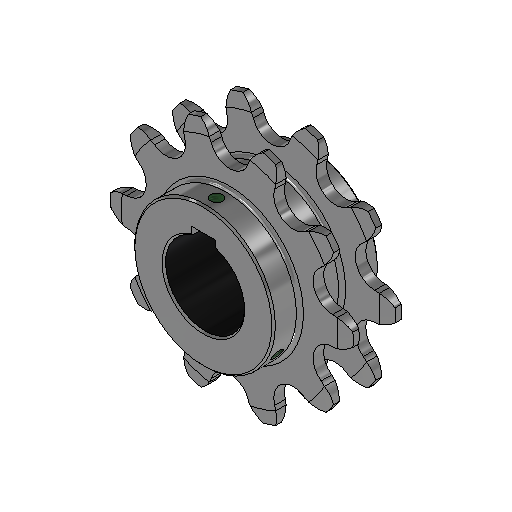
# Autodesk Inventor part: TL20240701-10110CV-016
Saved by Autodesk Inventor 2022.5 (Build 265521000, 521)
## iProperties
Category: DRIVE UNIT ASSY
Manager: 호상태
Company: 현대 트랜시스(대유)
Created: 2023-01-19
Part Number: TL20240701-10110CV-016
Project: SW PJT
Checked By: 김형민
Engr Approved By: 김시현
User Status: 2 x18
Material: S45C
Description: 0
Document SubType Name: Modeling
Mfg Approved By: 호상태
Designer: 박성규
Stock Number: 016
Density: 7.87 g/cm^3
Appearance: Plating Chrome
DETAIL: Coveryor Assembly
M/C TITLE: MEa/NEa차종 시트조립라인
SPECIFICATION: TL20221201-000000CV-006
DocNumber: 221118_Standard_v1
Folder: .\
VDS_Category: 엔지니어링
Detail Description: Processed products
Title: SPROCKET
Subject: SW차종 시트조립라인
Author: 박성규
Comments: RF2060 10NT
Revision Number: A
Autodesk Inventor part; units mm, degrees
ref_plane "YZ Plane" through (0, 0, 0) normal (1, 0, 0) x (0, 1, 0)
ref_plane "XZ Plane" through (0, 0, 0) normal (0, 1, 0) x (-1, 0, 0)
ref_plane "XY Plane" through (0, 0, 0) normal (0, 0, 1) x (1, 0, 0)
sketch "스케치8" plane through (0, 0, 0) normal (0, 0, 1) x (1, 0, 0)
  spline S0 degree 3 poles (-26.1552, 55.8268) (-26.2325, 56.5011) (-26.2682, 57.1822) (-26.249, 59.154) (-26.0828, 60.4461) (-25.5414, 62.6157) (-25.2309, 63.515) (-24.853, 64.3687) knots 0.551203 0.551203 0.551203 0.551203 0.748529 0.748529 1.122794 1.122794 1.401532 1.401532 1.401532 1.401532
  line L0 (-26.1552, 55.8268) -> (-26.2325, 56.5011) construction
  line L1 (-26.2325, 56.5011) -> (-26.2682, 57.1822) construction
  line L2 (-26.2682, 57.1822) -> (-26.249, 59.154) construction
  line L3 (-26.249, 59.154) -> (-26.0828, 60.4461) construction
  line L4 (-26.0828, 60.4461) -> (-25.5414, 62.6157) construction
  line L5 (-25.5414, 62.6157) -> (-25.2309, 63.515) construction
  line L6 (-25.2309, 63.515) -> (-24.853, 64.3687) construction
  arc A0 (-17.7285, 66.6836) -> (-24.853, 64.3687) centre (0, 0) ccw
  spline S1 degree 3 poles (-17.7285, 66.6836) (-16.921, 66.215) (-16.1411, 65.67) (-14.4279, 64.233) (-13.5339, 63.2854) (-12.3594, 61.7015) (-11.9879, 61.1294) (-11.6541, 60.5384) knots 4.560607 4.560607 4.560607 4.560607 4.839345 4.839345 5.213609 5.213609 5.410936 5.410936 5.410936 5.410936
  line L7 (-17.7285, 66.6836) -> (-16.921, 66.215) construction
  line L8 (-16.921, 66.215) -> (-16.1411, 65.67) construction
  line L9 (-16.1411, 65.67) -> (-14.4279, 64.233) construction
  line L10 (-14.4279, 64.233) -> (-13.5339, 63.2854) construction
  line L11 (-13.5339, 63.2854) -> (-12.3594, 61.7015) construction
  line L12 (-12.3594, 61.7015) -> (-11.9879, 61.1294) construction
  line L13 (-11.9879, 61.1294) -> (-11.6541, 60.5384) construction
  spline S2 degree 3 poles (11.6541, 60.5384) (11.9879, 61.1294) (12.3594, 61.7015) (13.5339, 63.2854) (14.4279, 64.233) (16.1411, 65.67) (16.921, 66.215) (17.7285, 66.6836) knots 0.551203 0.551203 0.551203 0.551203 0.748529 0.748529 1.122794 1.122794 1.401532 1.401532 1.401532 1.401532
  line L14 (11.6541, 60.5384) -> (11.9879, 61.1294) construction
  line L15 (11.9879, 61.1294) -> (12.3594, 61.7015) construction
  line L16 (12.3594, 61.7015) -> (13.5339, 63.2854) construction
  line L17 (13.5339, 63.2854) -> (14.4279, 64.233) construction
  line L18 (14.4279, 64.233) -> (16.1411, 65.67) construction
  line L19 (16.1411, 65.67) -> (16.921, 66.215) construction
  line L20 (16.921, 66.215) -> (17.7285, 66.6836) construction
  arc A1 (24.853, 64.3687) -> (17.7285, 66.6836) centre (0, 0) ccw
  spline S3 degree 3 poles (24.853, 64.3687) (25.2309, 63.515) (25.5414, 62.6157) (26.0828, 60.4461) (26.249, 59.154) (26.2682, 57.1822) (26.2325, 56.5011) (26.1552, 55.8268) knots 4.560607 4.560607 4.560607 4.560607 4.839345 4.839345 5.213609 5.213609 5.410936 5.410936 5.410936 5.410936
  line L21 (24.853, 64.3687) -> (25.2309, 63.515) construction
  line L22 (25.2309, 63.515) -> (25.5414, 62.6157) construction
  line L23 (25.5414, 62.6157) -> (26.0828, 60.4461) construction
  line L24 (26.0828, 60.4461) -> (26.249, 59.154) construction
  line L25 (26.249, 59.154) -> (26.2682, 57.1822) construction
  line L26 (26.2682, 57.1822) -> (26.2325, 56.5011) construction
  line L27 (26.2325, 56.5011) -> (26.1552, 55.8268) construction
  spline S4 degree 3 poles (45.012, 42.1265) (45.6294, 42.4084) (46.2662, 42.6528) (48.1474, 43.2439) (49.4276, 43.485) (51.6583, 43.6406) (52.6096, 43.6232) (53.5383, 43.5276) knots 0.551203 0.551203 0.551203 0.551203 0.748529 0.748529 1.122794 1.122794 1.401532 1.401532 1.401532 1.401532
  line L28 (45.012, 42.1265) -> (45.6294, 42.4084) construction
  line L29 (45.6294, 42.4084) -> (46.2662, 42.6528) construction
  line L30 (46.2662, 42.6528) -> (48.1474, 43.2439) construction
  line L31 (48.1474, 43.2439) -> (49.4276, 43.485) construction
  line L32 (49.4276, 43.485) -> (51.6583, 43.6406) construction
  line L33 (51.6583, 43.6406) -> (52.6096, 43.6232) construction
  line L34 (52.6096, 43.6232) -> (53.5383, 43.5276) construction
  arc A2 (57.9415, 37.4671) -> (53.5383, 43.5276) centre (0, 0) ccw
  spline S5 degree 3 poles (57.9415, 37.4671) (57.7454, 36.5544) (57.468, 35.6443) (56.6307, 33.5708) (56.0057, 32.4278) (54.8623, 30.8213) (54.433, 30.2912) (53.9742, 29.7912) knots 4.560607 4.560607 4.560607 4.560607 4.839345 4.839345 5.213609 5.213609 5.410936 5.410936 5.410936 5.410936
  line L35 (57.9415, 37.4671) -> (57.7454, 36.5544) construction
  line L36 (57.7454, 36.5544) -> (57.468, 35.6443) construction
  line L37 (57.468, 35.6443) -> (56.6307, 33.5708) construction
  line L38 (56.6307, 33.5708) -> (56.0057, 32.4278) construction
  line L39 (56.0057, 32.4278) -> (54.8623, 30.8213) construction
  line L40 (54.8623, 30.8213) -> (54.433, 30.2912) construction
  line L41 (54.433, 30.2912) -> (53.9742, 29.7912) construction
  spline S6 degree 3 poles (61.1768, 7.6237) (61.842, 7.4888) (62.5009, 7.3123) (64.3702, 6.6847) (65.5477, 6.1273) (67.4438, 4.942) (68.2031, 4.3688) (68.8983, 3.7456) knots 0.551203 0.551203 0.551203 0.551203 0.748529 0.748529 1.122794 1.122794 1.401532 1.401532 1.401532 1.401532
  line L42 (61.1768, 7.6237) -> (61.842, 7.4888) construction
  line L43 (61.842, 7.4888) -> (62.5009, 7.3123) construction
  line L44 (62.5009, 7.3123) -> (64.3702, 6.6847) construction
  line L45 (64.3702, 6.6847) -> (65.5477, 6.1273) construction
  line L46 (65.5477, 6.1273) -> (67.4438, 4.942) construction
  line L47 (67.4438, 4.942) -> (68.2031, 4.3688) construction
  line L48 (68.2031, 4.3688) -> (68.8983, 3.7456) construction
  arc A3 (68.8983, -3.7456) -> (68.8983, 3.7456) centre (0, 0) ccw
  spline S7 degree 3 poles (68.8983, -3.7456) (68.2031, -4.3688) (67.4438, -4.942) (65.5477, -6.1273) (64.3702, -6.6847) (62.5009, -7.3123) (61.842, -7.4888) (61.1768, -7.6237) knots 4.560607 4.560607 4.560607 4.560607 4.839345 4.839345 5.213609 5.213609 5.410936 5.410936 5.410936 5.410936
  line L49 (68.8983, -3.7456) -> (68.2031, -4.3688) construction
  line L50 (68.2031, -4.3688) -> (67.4438, -4.942) construction
  line L51 (67.4438, -4.942) -> (65.5477, -6.1273) construction
  line L52 (65.5477, -6.1273) -> (64.3702, -6.6847) construction
  line L53 (64.3702, -6.6847) -> (62.5009, -7.3123) construction
  line L54 (62.5009, -7.3123) -> (61.842, -7.4888) construction
  line L55 (61.842, -7.4888) -> (61.1768, -7.6237) construction
  spline S8 degree 3 poles (53.9742, -29.7912) (54.433, -30.2912) (54.8623, -30.8213) (56.0057, -32.4278) (56.6307, -33.5708) (57.468, -35.6443) (57.7454, -36.5544) (57.9415, -37.4671) knots 0.551203 0.551203 0.551203 0.551203 0.748529 0.748529 1.122794 1.122794 1.401532 1.401532 1.401532 1.401532
  line L56 (53.9742, -29.7912) -> (54.433, -30.2912) construction
  line L57 (54.433, -30.2912) -> (54.8623, -30.8213) construction
  line L58 (54.8623, -30.8213) -> (56.0057, -32.4278) construction
  line L59 (56.0057, -32.4278) -> (56.6307, -33.5708) construction
  line L60 (56.6307, -33.5708) -> (57.468, -35.6443) construction
  line L61 (57.468, -35.6443) -> (57.7454, -36.5544) construction
  line L62 (57.7454, -36.5544) -> (57.9415, -37.4671) construction
  arc A4 (53.5383, -43.5276) -> (57.9415, -37.4671) centre (0, 0) ccw
  spline S9 degree 3 poles (53.5383, -43.5276) (52.6096, -43.6232) (51.6583, -43.6406) (49.4276, -43.485) (48.1474, -43.2439) (46.2662, -42.6528) (45.6294, -42.4084) (45.012, -42.1265) knots 4.560607 4.560607 4.560607 4.560607 4.839345 4.839345 5.213609 5.213609 5.410936 5.410936 5.410936 5.410936
  line L63 (53.5383, -43.5276) -> (52.6096, -43.6232) construction
  line L64 (52.6096, -43.6232) -> (51.6583, -43.6406) construction
  line L65 (51.6583, -43.6406) -> (49.4276, -43.485) construction
  line L66 (49.4276, -43.485) -> (48.1474, -43.2439) construction
  line L67 (48.1474, -43.2439) -> (46.2662, -42.6528) construction
  line L68 (46.2662, -42.6528) -> (45.6294, -42.4084) construction
  line L69 (45.6294, -42.4084) -> (45.012, -42.1265) construction
  spline S10 degree 3 poles (26.1552, -55.8268) (26.2325, -56.5011) (26.2682, -57.1822) (26.249, -59.154) (26.0828, -60.4461) (25.5414, -62.6157) (25.2309, -63.515) (24.853, -64.3687) knots 0.551203 0.551203 0.551203 0.551203 0.748529 0.748529 1.122794 1.122794 1.401532 1.401532 1.401532 1.401532
  line L70 (26.1552, -55.8268) -> (26.2325, -56.5011) construction
  line L71 (26.2325, -56.5011) -> (26.2682, -57.1822) construction
  line L72 (26.2682, -57.1822) -> (26.249, -59.154) construction
  line L73 (26.249, -59.154) -> (26.0828, -60.4461) construction
  line L74 (26.0828, -60.4461) -> (25.5414, -62.6157) construction
  line L75 (25.5414, -62.6157) -> (25.2309, -63.515) construction
  line L76 (25.2309, -63.515) -> (24.853, -64.3687) construction
  arc A5 (17.7285, -66.6836) -> (24.853, -64.3687) centre (0, 0) ccw
  spline S11 degree 3 poles (17.7285, -66.6836) (16.921, -66.215) (16.1411, -65.67) (14.4279, -64.233) (13.5339, -63.2854) (12.3594, -61.7015) (11.9879, -61.1294) (11.6541, -60.5384) knots 4.560607 4.560607 4.560607 4.560607 4.839345 4.839345 5.213609 5.213609 5.410936 5.410936 5.410936 5.410936
  line L77 (17.7285, -66.6836) -> (16.921, -66.215) construction
  line L78 (16.921, -66.215) -> (16.1411, -65.67) construction
  line L79 (16.1411, -65.67) -> (14.4279, -64.233) construction
  line L80 (14.4279, -64.233) -> (13.5339, -63.2854) construction
  line L81 (13.5339, -63.2854) -> (12.3594, -61.7015) construction
  line L82 (12.3594, -61.7015) -> (11.9879, -61.1294) construction
  line L83 (11.9879, -61.1294) -> (11.6541, -60.5384) construction
  spline S12 degree 3 poles (-11.6541, -60.5384) (-11.9879, -61.1294) (-12.3594, -61.7015) (-13.5339, -63.2854) (-14.4279, -64.233) (-16.1411, -65.67) (-16.921, -66.215) (-17.7285, -66.6836) knots 0.551203 0.551203 0.551203 0.551203 0.748529 0.748529 1.122794 1.122794 1.401532 1.401532 1.401532 1.401532
  line L84 (-11.6541, -60.5384) -> (-11.9879, -61.1294) construction
  line L85 (-11.9879, -61.1294) -> (-12.3594, -61.7015) construction
  line L86 (-12.3594, -61.7015) -> (-13.5339, -63.2854) construction
  line L87 (-13.5339, -63.2854) -> (-14.4279, -64.233) construction
  line L88 (-14.4279, -64.233) -> (-16.1411, -65.67) construction
  line L89 (-16.1411, -65.67) -> (-16.921, -66.215) construction
  line L90 (-16.921, -66.215) -> (-17.7285, -66.6836) construction
  arc A6 (-24.853, -64.3687) -> (-17.7285, -66.6836) centre (0, 0) ccw
  spline S13 degree 3 poles (-24.853, -64.3687) (-25.2309, -63.515) (-25.5414, -62.6157) (-26.0828, -60.4461) (-26.249, -59.154) (-26.2682, -57.1822) (-26.2325, -56.5011) (-26.1552, -55.8268) knots 4.560607 4.560607 4.560607 4.560607 4.839345 4.839345 5.213609 5.213609 5.410936 5.410936 5.410936 5.410936
  line L91 (-24.853, -64.3687) -> (-25.2309, -63.515) construction
  line L92 (-25.2309, -63.515) -> (-25.5414, -62.6157) construction
  line L93 (-25.5414, -62.6157) -> (-26.0828, -60.4461) construction
  line L94 (-26.0828, -60.4461) -> (-26.249, -59.154) construction
  line L95 (-26.249, -59.154) -> (-26.2682, -57.1822) construction
  line L96 (-26.2682, -57.1822) -> (-26.2325, -56.5011) construction
  line L97 (-26.2325, -56.5011) -> (-26.1552, -55.8268) construction
  spline S14 degree 3 poles (-45.012, -42.1265) (-45.6294, -42.4084) (-46.2662, -42.6528) (-48.1474, -43.2439) (-49.4276, -43.485) (-51.6583, -43.6406) (-52.6096, -43.6232) (-53.5383, -43.5276) knots 0.551203 0.551203 0.551203 0.551203 0.748529 0.748529 1.122794 1.122794 1.401532 1.401532 1.401532 1.401532
  line L98 (-45.012, -42.1265) -> (-45.6294, -42.4084) construction
  line L99 (-45.6294, -42.4084) -> (-46.2662, -42.6528) construction
  line L100 (-46.2662, -42.6528) -> (-48.1474, -43.2439) construction
  line L101 (-48.1474, -43.2439) -> (-49.4276, -43.485) construction
  line L102 (-49.4276, -43.485) -> (-51.6583, -43.6406) construction
  line L103 (-51.6583, -43.6406) -> (-52.6096, -43.6232) construction
  line L104 (-52.6096, -43.6232) -> (-53.5383, -43.5276) construction
  arc A7 (-57.9415, -37.4671) -> (-53.5383, -43.5276) centre (0, 0) ccw
  spline S15 degree 3 poles (-57.9415, -37.4671) (-57.7454, -36.5544) (-57.468, -35.6443) (-56.6307, -33.5708) (-56.0057, -32.4278) (-54.8623, -30.8213) (-54.433, -30.2912) (-53.9742, -29.7912) knots 4.560607 4.560607 4.560607 4.560607 4.839345 4.839345 5.213609 5.213609 5.410936 5.410936 5.410936 5.410936
  line L105 (-57.9415, -37.4671) -> (-57.7454, -36.5544) construction
  line L106 (-57.7454, -36.5544) -> (-57.468, -35.6443) construction
  line L107 (-57.468, -35.6443) -> (-56.6307, -33.5708) construction
  line L108 (-56.6307, -33.5708) -> (-56.0057, -32.4278) construction
  line L109 (-56.0057, -32.4278) -> (-54.8623, -30.8213) construction
  line L110 (-54.8623, -30.8213) -> (-54.433, -30.2912) construction
  line L111 (-54.433, -30.2912) -> (-53.9742, -29.7912) construction
  spline S16 degree 3 poles (-53.9742, 29.7912) (-54.433, 30.2912) (-54.8623, 30.8213) (-56.0057, 32.4278) (-56.6307, 33.5708) (-57.468, 35.6443) (-57.7454, 36.5544) (-57.9415, 37.4671) knots 0.551203 0.551203 0.551203 0.551203 0.748529 0.748529 1.122794 1.122794 1.401532 1.401532 1.401532 1.401532
  line L112 (-53.9742, 29.7912) -> (-54.433, 30.2912) construction
  line L113 (-54.433, 30.2912) -> (-54.8623, 30.8213) construction
  line L114 (-54.8623, 30.8213) -> (-56.0057, 32.4278) construction
  line L115 (-56.0057, 32.4278) -> (-56.6307, 33.5708) construction
  line L116 (-56.6307, 33.5708) -> (-57.468, 35.6443) construction
  line L117 (-57.468, 35.6443) -> (-57.7454, 36.5544) construction
  line L118 (-57.7454, 36.5544) -> (-57.9415, 37.4671) construction
  arc A8 (-53.5383, 43.5276) -> (-57.9415, 37.4671) centre (0, 0) ccw
  spline S17 degree 3 poles (-53.5383, 43.5276) (-52.6096, 43.6232) (-51.6583, 43.6406) (-49.4276, 43.485) (-48.1474, 43.2439) (-46.2662, 42.6528) (-45.6294, 42.4084) (-45.012, 42.1265) knots 4.560607 4.560607 4.560607 4.560607 4.839345 4.839345 5.213609 5.213609 5.410936 5.410936 5.410936 5.410936
  line L119 (-53.5383, 43.5276) -> (-52.6096, 43.6232) construction
  line L120 (-52.6096, 43.6232) -> (-51.6583, 43.6406) construction
  line L121 (-51.6583, 43.6406) -> (-49.4276, 43.485) construction
  line L122 (-49.4276, 43.485) -> (-48.1474, 43.2439) construction
  line L123 (-48.1474, 43.2439) -> (-46.2662, 42.6528) construction
  line L124 (-46.2662, 42.6528) -> (-45.6294, 42.4084) construction
  line L125 (-45.6294, 42.4084) -> (-45.012, 42.1265) construction
  spline S18 degree 3 poles (-68.8983, 3.7456) (-68.2031, 4.3688) (-67.4438, 4.942) (-65.5477, 6.1273) (-64.3702, 6.6847) (-62.5009, 7.3123) (-61.842, 7.4888) (-61.1768, 7.6237) knots 4.560607 4.560607 4.560607 4.560607 4.839345 4.839345 5.213609 5.213609 5.410936 5.410936 5.410936 5.410936
  line L126 (-68.8983, 3.7456) -> (-68.2031, 4.3688) construction
  line L127 (-68.2031, 4.3688) -> (-67.4438, 4.942) construction
  line L128 (-67.4438, 4.942) -> (-65.5477, 6.1273) construction
  line L129 (-65.5477, 6.1273) -> (-64.3702, 6.6847) construction
  line L130 (-64.3702, 6.6847) -> (-62.5009, 7.3123) construction
  line L131 (-62.5009, 7.3123) -> (-61.842, 7.4888) construction
  line L132 (-61.842, 7.4888) -> (-61.1768, 7.6237) construction
  spline S19 degree 3 poles (-61.1768, -7.6237) (-61.842, -7.4888) (-62.5009, -7.3123) (-64.3702, -6.6847) (-65.5477, -6.1273) (-67.4438, -4.942) (-68.2031, -4.3688) (-68.8983, -3.7456) knots 0.551203 0.551203 0.551203 0.551203 0.748529 0.748529 1.122794 1.122794 1.401532 1.401532 1.401532 1.401532
  line L133 (-61.1768, -7.6237) -> (-61.842, -7.4888) construction
  line L134 (-61.842, -7.4888) -> (-62.5009, -7.3123) construction
  line L135 (-62.5009, -7.3123) -> (-64.3702, -6.6847) construction
  line L136 (-64.3702, -6.6847) -> (-65.5477, -6.1273) construction
  line L137 (-65.5477, -6.1273) -> (-67.4438, -4.942) construction
  line L138 (-67.4438, -4.942) -> (-68.2031, -4.3688) construction
  line L139 (-68.2031, -4.3688) -> (-68.8983, -3.7456) construction
  arc A9 (-68.8983, 3.7456) -> (-68.8983, -3.7456) centre (0, 0) ccw
  arc A10 (45.012, 42.1265) -> (42.7702, 40.8837) centre (51.8522, 27.1447) ccw
  arc A11 (11.6541, 60.5384) -> (10.571, 58.2153) centre (25.9941, 52.4385) ccw
  arc A12 (-26.1552, 55.8268) -> (-25.666, 53.3106) centre (-9.7929, 57.7026) ccw
  arc A13 (-53.9742, 29.7912) -> (-52.0994, 28.0431) centre (-41.8394, 40.9262) ccw
  arc A14 (-45.012, -42.1265) -> (-42.7702, -40.8837) centre (-51.8522, -27.1447) ccw
  arc A15 (-11.6541, -60.5384) -> (-10.571, -58.2153) centre (-25.9941, -52.4385) ccw
  arc A16 (26.1552, -55.8268) -> (25.666, -53.3106) centre (9.7929, -57.7026) ccw
  arc A17 (53.9742, -29.7912) -> (52.0994, -28.0431) centre (41.8394, -40.9262) ccw
  arc A18 (61.1768, 7.6237) -> (58.6326, 7.9359) centre (57.9046, -8.5175) ccw
  arc A19 (-58.6326, 7.9359) -> (-61.1768, 7.6237) centre (-57.9046, -8.5175) ccw
  arc A20 (-58.6326, 7.9359) -> (-52.0994, 28.0431) centre (-58.6326, 19.0509) ccw
  arc A21 (-42.7702, 40.8837) -> (-45.012, 42.1265) centre (-51.8522, 27.1447) ccw
  arc A22 (-42.7702, 40.8837) -> (-25.666, 53.3106) centre (-36.237, 49.8759) ccw
  arc A23 (-10.571, 58.2153) -> (-11.6541, 60.5384) centre (-25.9941, 52.4385) ccw
  arc A24 (-10.571, 58.2153) -> (10.571, 58.2153) centre (0, 61.65) ccw
  arc A25 (25.666, 53.3106) -> (26.1552, 55.8268) centre (9.7929, 57.7026) ccw
  arc A26 (25.666, 53.3106) -> (42.7702, 40.8837) centre (36.237, 49.8759) ccw
  arc A27 (52.0994, 28.0431) -> (53.9742, 29.7912) centre (41.8394, 40.9262) ccw
  arc A28 (52.0994, 28.0431) -> (58.6326, 7.9359) centre (58.6326, 19.0509) ccw
  arc A29 (58.6326, -7.9359) -> (61.1768, -7.6237) centre (57.9046, 8.5175) ccw
  arc A30 (58.6326, -7.9359) -> (52.0994, -28.0431) centre (58.6326, -19.0509) ccw
  arc A31 (42.7702, -40.8837) -> (45.012, -42.1265) centre (51.8522, -27.1447) ccw
  arc A32 (42.7702, -40.8837) -> (25.666, -53.3106) centre (36.237, -49.8759) ccw
  arc A33 (10.571, -58.2153) -> (11.6541, -60.5384) centre (25.9941, -52.4385) ccw
  arc A34 (10.571, -58.2153) -> (-10.571, -58.2153) centre (0, -61.65) ccw
  arc A35 (-25.666, -53.3106) -> (-26.1552, -55.8268) centre (-9.7929, -57.7026) ccw
  arc A36 (-25.666, -53.3106) -> (-42.7702, -40.8837) centre (-36.237, -49.8759) ccw
  arc A37 (-52.0994, -28.0431) -> (-53.9742, -29.7912) centre (-41.8394, -40.9262) ccw
  arc A38 (-52.0994, -28.0431) -> (-58.6326, -7.9359) centre (-58.6326, -19.0509) ccw
  arc A39 (-61.1768, -7.6237) -> (-58.6326, -7.9359) centre (-57.9046, 8.5175) ccw
  point P0 (0, 0)
  constraints: 80 point on circle, 40 centre point, 1 coincident, 60 other
extrude "돌출3" add sketch "스케치8" along normal blind 6
sketch "스케치9" plane through (0, 0, 6) normal (0, 0, 1) x (1, 0, 0)
  arc A0 (-17.7285, 66.6836) -> (-24.853, 64.3687) centre (0, 0) ccw construction
  circle A1 centre (0, 0) radius 40
  dimension "d40" = 80
  constraints: 1 centre point, 1 coincident
  measures "d40" diameter of A1
extrude "돌출4" add sketch "스케치9" along normal blind 18
sketch "스케치10" plane through (0, 0, 24) normal (0, 0, 1) x (1, 0, 0)
  arc A0 (-42.7702, 40.8837) -> (-25.666, 53.3106) centre (-36.237, 49.8759) ccw projected
  spline S0 degree 3 poles (-45.012, 42.1265) (-45.6294, 42.4084) (-46.2662, 42.6528) (-48.1474, 43.2439) (-49.4276, 43.485) (-51.6583, 43.6406) (-52.6096, 43.6232) (-53.5383, 43.5276) knots 0 0 0 0 0.232059 0.232059 0.6722 0.6722 1 1 1 1 projected
  arc A1 (-42.7702, 40.8837) -> (-45.012, 42.1265) centre (-51.8522, 27.1447) ccw projected
  arc A2 (-42.7702, 40.8837) -> (-25.666, 53.3106) centre (-36.237, 49.8759) ccw projected
  arc A3 (-26.1552, 55.8268) -> (-25.666, 53.3106) centre (-9.7929, 57.7026) ccw projected
  spline S1 degree 3 poles (-24.853, 64.3687) (-25.2309, 63.515) (-25.5414, 62.6157) (-26.0828, 60.4461) (-26.249, 59.154) (-26.2682, 57.1822) (-26.2325, 56.5011) (-26.1552, 55.8268) knots 0 0 0 0 0.3278 0.3278 0.767941 0.767941 1 1 1 1 projected
  arc A4 (-17.7285, 66.6836) -> (-24.853, 64.3687) centre (0, 0) ccw projected
  spline S2 degree 3 poles (-11.6541, 60.5384) (-11.9879, 61.1294) (-12.3594, 61.7015) (-13.5339, 63.2854) (-14.4279, 64.233) (-16.1411, 65.67) (-16.921, 66.215) (-17.7285, 66.6836) knots 0 0 0 0 0.232059 0.232059 0.6722 0.6722 1 1 1 1 projected
  arc A5 (-10.571, 58.2153) -> (-11.6541, 60.5384) centre (-25.9941, 52.4385) ccw projected
  arc A6 (-10.571, 58.2153) -> (10.571, 58.2153) centre (0, 61.65) ccw projected
  arc A7 (11.6541, 60.5384) -> (10.571, 58.2153) centre (25.9941, 52.4385) ccw projected
  spline S3 degree 3 poles (17.7285, 66.6836) (16.921, 66.215) (16.1411, 65.67) (14.4279, 64.233) (13.5339, 63.2854) (12.3594, 61.7015) (11.9879, 61.1294) (11.6541, 60.5384) knots 0 0 0 0 0.3278 0.3278 0.767941 0.767941 1 1 1 1 projected
  arc A8 (24.853, 64.3687) -> (17.7285, 66.6836) centre (0, 0) ccw projected
  spline S4 degree 3 poles (26.1552, 55.8268) (26.2325, 56.5011) (26.2682, 57.1822) (26.249, 59.154) (26.0828, 60.4461) (25.5414, 62.6157) (25.2309, 63.515) (24.853, 64.3687) knots 0 0 0 0 0.232059 0.232059 0.6722 0.6722 1 1 1 1 projected
  arc A9 (25.666, 53.3106) -> (26.1552, 55.8268) centre (9.7929, 57.7026) ccw projected
  arc A10 (25.666, 53.3106) -> (42.7702, 40.8837) centre (36.237, 49.8759) ccw projected
  arc A11 (45.012, 42.1265) -> (42.7702, 40.8837) centre (51.8522, 27.1447) ccw projected
  spline S5 degree 3 poles (53.5383, 43.5276) (52.6096, 43.6232) (51.6583, 43.6406) (49.4276, 43.485) (48.1474, 43.2439) (46.2662, 42.6528) (45.6294, 42.4084) (45.012, 42.1265) knots 0 0 0 0 0.3278 0.3278 0.767941 0.767941 1 1 1 1 projected
  arc A12 (57.9415, 37.4671) -> (53.5383, 43.5276) centre (0, 0) ccw projected
  spline S6 degree 3 poles (53.9742, 29.7912) (54.433, 30.2912) (54.8623, 30.8213) (56.0057, 32.4278) (56.6307, 33.5708) (57.468, 35.6443) (57.7454, 36.5544) (57.9415, 37.4671) knots 0 0 0 0 0.232059 0.232059 0.6722 0.6722 1 1 1 1 projected
  arc A13 (52.0994, 28.0431) -> (53.9742, 29.7912) centre (41.8394, 40.9262) ccw projected
  arc A14 (52.0994, 28.0431) -> (58.6326, 7.9359) centre (58.6326, 19.0509) ccw projected
  arc A15 (61.1768, 7.6237) -> (58.6326, 7.9359) centre (57.9046, -8.5175) ccw projected
  spline S7 degree 3 poles (68.8983, 3.7456) (68.2031, 4.3688) (67.4438, 4.942) (65.5477, 6.1273) (64.3702, 6.6847) (62.5009, 7.3123) (61.842, 7.4888) (61.1768, 7.6237) knots 0 0 0 0 0.3278 0.3278 0.767941 0.767941 1 1 1 1 projected
  arc A16 (68.8983, -3.7456) -> (68.8983, 3.7456) centre (0, 0) ccw projected
  spline S8 degree 3 poles (61.1768, -7.6237) (61.842, -7.4888) (62.5009, -7.3123) (64.3702, -6.6847) (65.5477, -6.1273) (67.4438, -4.942) (68.2031, -4.3688) (68.8983, -3.7456) knots 0 0 0 0 0.232059 0.232059 0.6722 0.6722 1 1 1 1 projected
  arc A17 (58.6326, -7.9359) -> (61.1768, -7.6237) centre (57.9046, 8.5175) ccw projected
  arc A18 (58.6326, -7.9359) -> (52.0994, -28.0431) centre (58.6326, -19.0509) ccw projected
  arc A19 (53.9742, -29.7912) -> (52.0994, -28.0431) centre (41.8394, -40.9262) ccw projected
  spline S9 degree 3 poles (57.9415, -37.4671) (57.7454, -36.5544) (57.468, -35.6443) (56.6307, -33.5708) (56.0057, -32.4278) (54.8623, -30.8213) (54.433, -30.2912) (53.9742, -29.7912) knots 0 0 0 0 0.3278 0.3278 0.767941 0.767941 1 1 1 1 projected
  arc A20 (53.5383, -43.5276) -> (57.9415, -37.4671) centre (0, 0) ccw projected
  spline S10 degree 3 poles (45.012, -42.1265) (45.6294, -42.4084) (46.2662, -42.6528) (48.1474, -43.2439) (49.4276, -43.485) (51.6583, -43.6406) (52.6096, -43.6232) (53.5383, -43.5276) knots 0 0 0 0 0.232059 0.232059 0.6722 0.6722 1 1 1 1 projected
  arc A21 (42.7702, -40.8837) -> (45.012, -42.1265) centre (51.8522, -27.1447) ccw projected
  arc A22 (42.7702, -40.8837) -> (25.666, -53.3106) centre (36.237, -49.8759) ccw projected
  arc A23 (26.1552, -55.8268) -> (25.666, -53.3106) centre (9.7929, -57.7026) ccw projected
  spline S11 degree 3 poles (24.853, -64.3687) (25.2309, -63.515) (25.5414, -62.6157) (26.0828, -60.4461) (26.249, -59.154) (26.2682, -57.1822) (26.2325, -56.5011) (26.1552, -55.8268) knots 0 0 0 0 0.3278 0.3278 0.767941 0.767941 1 1 1 1 projected
  arc A24 (17.7285, -66.6836) -> (24.853, -64.3687) centre (0, 0) ccw projected
  spline S12 degree 3 poles (11.6541, -60.5384) (11.9879, -61.1294) (12.3594, -61.7015) (13.5339, -63.2854) (14.4279, -64.233) (16.1411, -65.67) (16.921, -66.215) (17.7285, -66.6836) knots 0 0 0 0 0.232059 0.232059 0.6722 0.6722 1 1 1 1 projected
  arc A25 (10.571, -58.2153) -> (11.6541, -60.5384) centre (25.9941, -52.4385) ccw projected
  arc A26 (10.571, -58.2153) -> (-10.571, -58.2153) centre (0, -61.65) ccw projected
  arc A27 (-11.6541, -60.5384) -> (-10.571, -58.2153) centre (-25.9941, -52.4385) ccw projected
  spline S13 degree 3 poles (-17.7285, -66.6836) (-16.921, -66.215) (-16.1411, -65.67) (-14.4279, -64.233) (-13.5339, -63.2854) (-12.3594, -61.7015) (-11.9879, -61.1294) (-11.6541, -60.5384) knots 0 0 0 0 0.3278 0.3278 0.767941 0.767941 1 1 1 1 projected
  arc A28 (-24.853, -64.3687) -> (-17.7285, -66.6836) centre (0, 0) ccw projected
  spline S14 degree 3 poles (-26.1552, -55.8268) (-26.2325, -56.5011) (-26.2682, -57.1822) (-26.249, -59.154) (-26.0828, -60.4461) (-25.5414, -62.6157) (-25.2309, -63.515) (-24.853, -64.3687) knots 0 0 0 0 0.232059 0.232059 0.6722 0.6722 1 1 1 1 projected
  arc A29 (-25.666, -53.3106) -> (-26.1552, -55.8268) centre (-9.7929, -57.7026) ccw projected
  arc A30 (-25.666, -53.3106) -> (-42.7702, -40.8837) centre (-36.237, -49.8759) ccw projected
  arc A31 (-45.012, -42.1265) -> (-42.7702, -40.8837) centre (-51.8522, -27.1447) ccw projected
  spline S15 degree 3 poles (-53.5383, -43.5276) (-52.6096, -43.6232) (-51.6583, -43.6406) (-49.4276, -43.485) (-48.1474, -43.2439) (-46.2662, -42.6528) (-45.6294, -42.4084) (-45.012, -42.1265) knots 0 0 0 0 0.3278 0.3278 0.767941 0.767941 1 1 1 1 projected
  arc A32 (-57.9415, -37.4671) -> (-53.5383, -43.5276) centre (0, 0) ccw projected
  spline S16 degree 3 poles (-53.9742, -29.7912) (-54.433, -30.2912) (-54.8623, -30.8213) (-56.0057, -32.4278) (-56.6307, -33.5708) (-57.468, -35.6443) (-57.7454, -36.5544) (-57.9415, -37.4671) knots 0 0 0 0 0.232059 0.232059 0.6722 0.6722 1 1 1 1 projected
  arc A33 (-52.0994, -28.0431) -> (-53.9742, -29.7912) centre (-41.8394, -40.9262) ccw projected
  arc A34 (-52.0994, -28.0431) -> (-58.6326, -7.9359) centre (-58.6326, -19.0509) ccw projected
  arc A35 (-61.1768, -7.6237) -> (-58.6326, -7.9359) centre (-57.9046, 8.5175) ccw projected
  spline S17 degree 3 poles (-68.8983, -3.7456) (-68.2031, -4.3688) (-67.4438, -4.942) (-65.5477, -6.1273) (-64.3702, -6.6847) (-62.5009, -7.3123) (-61.842, -7.4888) (-61.1768, -7.6237) knots 0 0 0 0 0.3278 0.3278 0.767941 0.767941 1 1 1 1 projected
  arc A36 (-68.8983, 3.7456) -> (-68.8983, -3.7456) centre (0, 0) ccw projected
  spline S18 degree 3 poles (-61.1768, 7.6237) (-61.842, 7.4888) (-62.5009, 7.3123) (-64.3702, 6.6847) (-65.5477, 6.1273) (-67.4438, 4.942) (-68.2031, 4.3688) (-68.8983, 3.7456) knots 0 0 0 0 0.232059 0.232059 0.6722 0.6722 1 1 1 1 projected
  arc A37 (-58.6326, 7.9359) -> (-61.1768, 7.6237) centre (-57.9046, -8.5175) ccw projected
  arc A38 (-58.6326, 7.9359) -> (-52.0994, 28.0431) centre (-58.6326, 19.0509) ccw projected
  arc A39 (-53.9742, 29.7912) -> (-52.0994, 28.0431) centre (-41.8394, 40.9262) ccw projected
  spline S19 degree 3 poles (-57.9415, 37.4671) (-57.7454, 36.5544) (-57.468, 35.6443) (-56.6307, 33.5708) (-56.0057, 32.4278) (-54.8623, 30.8213) (-54.433, 30.2912) (-53.9742, 29.7912) knots 0 0 0 0 0.3278 0.3278 0.767941 0.767941 1 1 1 1 projected
  arc A40 (-53.5383, 43.5276) -> (-57.9415, 37.4671) centre (0, 0) ccw projected
  point P0 (-25.666, 53.3106)
  point P1 (-42.7702, 40.8837)
  constraints: 20 other
extrude "돌출5" add sketch "스케치10" along normal blind 6
sketch "스케치11" plane through (0, 0, 30) normal (0, 0, 1) x (1, 0, 0)
  arc A0 (-17.7285, 66.6836) -> (-24.853, 64.3687) centre (0, 0) ccw construction
  circle A1 centre (0, 0) radius 40
  dimension "d45" = 80
  constraints: 1 centre point, 1 coincident
  measures "d45" diameter of A1
extrude "돌출6" add sketch "스케치11" along normal blind 15
sketch "스케치12" plane through (0, 0, 0) normal (0, 1, 0) x (-1, 0, 0)
  line L0 (69, 0) -> (69, 1.3)
  line L1 (69, 1.3) -> (61.65, 0)
  line L2 (61.65, 0) -> (69, 0)
  line L3 (69, 4.7) -> (69, 6)
  line L4 (69, 6) -> (61.65, 6)
  line L5 (61.65, 6) -> (69, 4.7)
  line L6 (69, 24) -> (61.65, 24)
  line L7 (61.65, 24) -> (69, 25.3)
  line L8 (69, 25.3) -> (69, 24)
  line L9 (69, 28.7) -> (69, 30)
  line L10 (69, 30) -> (61.65, 30)
  line L11 (61.65, 30) -> (69, 28.7)
  line L12 (69, 0) -> (69, 6) construction
  line L13 (61.1768, 30) -> (68.8983, 30) construction
  line L14 (61.1768, 24) -> (68.8983, 24) construction
  line L15 (61.1768, 6) -> (68.8983, 6) construction
  line L16 (61.1768, 0) -> (68.8983, 0) construction
  line L17 (0, 0) -> (0, 55.1303)
  dimension "d48" = 7.35
  dimension "d49" = 1.3
  dimension "d50" = 1.3
  dimension "d51" = 1.3
  dimension "d52" = 1.3
  constraints: 26 end point, 7 collinear, 4 perpendicular, 3 vertical, 3 vertical alignment, 2 point on line, 1 horizontal
  measures "d48" distance of L1.end L0.start
  measures "d49" distance of L0.start L0.end
  measures "d50" distance of L3.start L3.end
  measures "d51" distance of L7.end L6.start
  measures "d52" distance of L9.start L9.end
revolve "회전1" cut sketch "스케치12" angle 360 about axis through (0, 0, 0) along (0, 0, 1)
sketch "스케치13" plane through (0, 0, 45) normal (0, 0, 1) x (1, 0, 0)
  circle A0 centre (0, 0) radius 40 construction
  point P0 (0, 0)
  constraints: 1 coincident
hole "구멍3" at (0, 0, 45) direction (0, 0, -1) diameter 45 end through all
sketch "스케치14" plane through (0, 0, 45) normal (0, 0, 1) x (1, 0, 0)
  circle A0 centre (0, 0) radius 22.5 construction
  line L0 (-7, 26.3) -> (7, 26.3)
  line L1 (7, 26.3) -> (7, 16.3)
  line L2 (7, 16.3) -> (-7, 16.3)
  line L3 (-7, 16.3) -> (-7, 26.3)
  line L4 (-7, 26.3) -> (7, 16.3) construction
  line L5 (7, 26.3) -> (-7, 16.3) construction
  point P0 (0, 21.3)
  point P1 (0, 21.3)
  dimension "d61" = 14
  dimension "d62" = 26.3
  dimension "d63" = 10
  constraints: 12 end point, 3 midpoint, 2 parallel, 1 horizontal, 1 perpendicular, 1 vertical alignment
  measures "d61" distance of L0.start L0.end
  measures "d62" distance from line of A0.centre L0
  measures "d63" distance of L0.end L1.end
extrude "돌출7" cut sketch "스케치14" against normal blind 50
sketch "스케치15" plane through (0, 0, 0) normal (0, 0, -1) x (-1, 0, 0)
  line L0 (-7, 21.3834) -> (-7, 26.3) projected
  line L1 (-7, 26.3) -> (7, 26.3) projected
  line L2 (7, 26.3) -> (7, 21.3834) projected
  arc A0 (-7, 21.3834) -> (7, 21.3834) centre (0, 0) ccw projected
  circle A1 centre (0, 0) radius 40
  dimension "d73" = 80
  constraints: 1 centre point, 1 coincident
  measures "d73" diameter of A1
extrude "돌출8" add sketch "스케치15" along normal blind 15
chamfer "모따기3" distance 1 angle 45 4 edges at (0, -22.5, 45) (-40, 0, 45) (40, 0, -15) (0, -22.5, -15)
fillet "모깎기3" radius 2 4 edges at (40, 0, 0) (-40, 0, 6) (-40, 0, 24) (-40, 0, 30)
sketch "스케치16" plane through (0, 0, 0) normal (0, 1, 0) x (-1, 0, 0)
  line L0 (-39, 45) -> (39, 45) construction
  line L1 (39, -15) -> (-39, -15) construction
  line L2 (-10.571, 0) -> (10.571, 0) construction
  point P0 (0, 0)
  point P1 (0, -7.5)
  point P2 (0, 37.5)
  point P3 (0, 0)
  point P4 (0, 0)
  dimension "d80" = 7.5
  dimension "d81" = 7.5
  constraints: 2 midpoint, 2 vertical alignment
  measures "d80" distance from line of L0 point (0, 37.5)
  measures "d81" distance from line of L1 point (0, -7.5)
hole "구멍4" at (0, 0, -7.5) at (0, 0, 37.5) direction (0, 1, 0) diameter 6.647 end through all start extended yes thread size "M8x1.25" class "6H" standard "ISO Metric profile"
pattern_circular "원형 패턴1" count 2 over 120 about axis through (0, 0, 0) along (0, 0, -1) of "구멍4"
sketch "스케치17" plane through (22.7765, -13.15, -7.5) normal (0.8660254, -0.5, 0) x (0, 0, -1)
  circle A0 centre (0, 0) radius 3.3235 construction
  circle A1 centre (-45, 0) radius 3.3235 construction
  point P0 (-7.5, 0)
  point P1 (0, 0)
  point P2 (-45, 0)
  constraints: 2 coincident
hole "구멍5" at (22.7765, -13.15, -7.5) at (22.7765, -13.15, 37.5) direction (-0.8660254, 0.5, 0) diameter 6.647 end up to face face through (0, 0, -152.1193) facing (0, 0, 1) round with radius 22.5 far side no start extended yes thread size "M8x1.25" class "6H" standard "ISO Metric profile"
